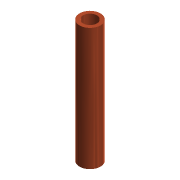
# Autodesk Inventor part: 17-0028-0104
Saved by Autodesk Inventor 2016 SP2 (Build 200236200, 236)
## iProperties
Category: IOP
Company: Universiteit van Amsterdam
Created: 2017-12-13
Part Number: 17-0028-0104
Material: Copper
Document SubType Name: Modeling
Designer: Daan Giesen
Density: 8.94 g/cm^3
Appearance: Copper - Satin
Project: Digital PID Loop
Cost Center: 17-0028
User Status: Work in Progress
Authority: Reichsöllner, Lukas
Description: Cooling tube
Mass: 5.61717 g
Surface Area: 12.8805 cm^2
Volume: 0.628319 cm^3
Author: Daan Giesen
Title: Digital PID Loop
Revision Number: A
Autodesk Inventor part; units mm, degrees
ref_plane "YZ Plane" through (0, 0, 0) normal (1, 0, 0) x (0, 1, 0)
ref_plane "XZ Plane" through (0, 0, 0) normal (0, 1, 0) x (-1, 0, 0)
ref_plane "XY Plane" through (0, 0, 0) normal (0, 0, 1) x (1, 0, 0)
sketch "Sketch1" plane through (0, 0, 0) normal (0, 0, 1) x (1, 0, 0)
  line L0 (0, 4.2) -> (0, -4.2) construction
  line L1 (-4.2, 0) -> (4.2, 0) construction
  circle A0 centre (0, 0) radius 2
  circle A1 centre (0, 0) radius 3
  dimension "d4" = 6
  dimension "d5" = 4
  constraints: 2 centre point, 2 coincident
  measures "d4" diameter of A1
  measures "d5" diameter of A0
extrude "Extrusion3" add sketch "Sketch1" along normal blind 40
body "Solid3"
